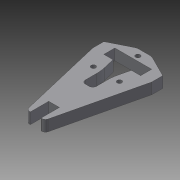
# Autodesk Inventor part: Vert Moto Mount skinny
Saved by Autodesk Inventor 2015 (Build 190159000, 159)
## iProperties
Created: 2012-05-11
Part Number: Vert Moto Mount skinny
Material: Generic
Document SubType Name: Modeling
Designer: user
Density: 1 g/cm^3
Appearance: Default
Author: user
Autodesk Inventor part; units mm, degrees
ref_plane "YZ Plane" through (0, 0, 0) normal (1, 0, 0) x (0, 1, 0)
ref_plane "XZ Plane" through (0, 0, 0) normal (0, 1, 0) x (-1, 0, 0)
ref_plane "XY Plane" through (0, 0, 0) normal (0, 0, 1) x (1, 0, 0)
sketch "Sketch1" plane through (0, 0, 0) normal (0, 0, 1) x (1, 0, 0)
  circle A0 centre (0, 35.5) radius 10 construction
  line L0 (-2.9, -10) -> (-2.9, 0)
  line L1 (-2.9, 0) -> (2.9, 0)
  line L2 (2.9, 0) -> (2.9, -10)
  line L3 (-3.3173, -10) -> (-2.9, -10)
  line L4 (2.9, -10) -> (3.3173, -10)
  circle A1 centre (-7.0711, 28.4289) radius 1.25
  circle A2 centre (7.0711, 28.4289) radius 1.25
  circle A3 centre (0, 45.5) radius 1.25
  line L5 (-16, 37) -> (-16, 43)
  line L6 (16, 37) -> (16, 43)
  line L7 (-5.2638, -8.4597) -> (-16, 37)
  line L8 (5.2638, -8.4597) -> (16, 37)
  line L9 (-16, 43) -> (-4.8446, 48.5777)
  line L10 (-3.0557, 49) -> (3.0557, 49)
  line L11 (4.8446, 48.5777) -> (16, 43)
  arc A4 (-3.0557, 49) -> (-4.8446, 48.5777) centre (-3.0557, 45) ccw
  arc A5 (4.8446, 48.5777) -> (3.0557, 49) centre (3.0557, 45) ccw
  line L12 (0, 49) -> (0, 0) construction
  line L13 (-7.0711, 28.4289) -> (0, 35.5) construction
  line L14 (0, 35.5) -> (7.0711, 28.4289) construction
  arc A6 (-5.2638, -8.4597) -> (-3.3173, -10) centre (-3.3173, -8) ccw
  arc A7 (3.3173, -10) -> (5.2638, -8.4597) centre (3.3173, -8) ccw
  circle A8 centre (0, 35.5) radius 15.25 construction
  point P0 (0, 43)
  point P1 (4.9, -10)
  point P2 (-4.9, -10)
  point P3 (0, 43)
  point P4 (-4, 49)
  point P5 (4, 49)
  dimension "d69" = 20
  dimension "d88" = 5.8
  dimension "d95" = 2
  dimension "d96" = 2
  dimension "d97" = 10
  dimension "d98" = 10
  dimension "d109" = 43
  dimension "d112" = 2.5
  dimension "d113" = 2.5
  dimension "d114" = 2.5
  dimension "d123" = 32
  dimension "d126" = 8
  dimension "d127" = 4
  dimension "d144" = 16
  dimension "d145" = 35.5
  dimension "d153" = 6
  dimension "d155" = 6
  dimension "d156" = 135
  dimension "d163" = 2
  dimension "d169" = 30.5
  constraints: 30 end point, 12 point on circle, 9 centre point, 8 point on line, 8 tangent, 5 coincident, 5 perpendicular, 4 horizontal alignment, 4 vertical alignment, 2 equal length, 2 equal radius, 2 midpoint, 1 horizontal, 1 vertical
  measures "d69" diameter of A0
  measures "d88" distance of L0.end L1.end
  measures "d95" distance of point (-4.9, -10) L0.start
  measures "d96" distance of L2.end point (4.9, -10)
  measures "d97" distance between parallel lines of L3 L1
  measures "d98" distance between parallel lines of L1 L4
  measures "d109" distance from line of L1 point (0, 43)
  measures "d112" diameter of A2
  measures "d113" diameter of A1
  measures "d114" diameter of A3
  measures "d123" distance between parallel lines of L6 L5
  measures "d126" distance of point (-4, 49) point (4, 49)
  measures "d127" radius of A4
  measures "d144" distance from line of L13.end L6
  measures "d145" distance from line of L1 L13.end
  measures "d153" distance of L5.start L5.end
  measures "d155" distance from line of L5.end L10
  measures "d156" angle of L12 L13
  measures "d163" radius of A6
  measures "d169" diameter of A8
extrude "Extrusion7" add sketch "Sketch1" along normal blind 6
sketch "Sketch3" plane through (0, 0, 6) normal (0, 0, 1) x (1, 0, 0)
  line L0 (16, 37) -> (16, 43) projected
  line L1 (-16, 43) -> (-16, 37) projected
  line L2 (-10, 43) -> (10, 43)
  line L3 (10, 43) -> (10, 37)
  line L4 (-10, 37) -> (-10, 43)
  line L5 (10, 37) -> (5, 37)
  line L6 (-5, 37) -> (-10, 37)
  line L7 (5.2638, -8.4597) -> (16, 37) projected
  line L8 (-16, 37) -> (-5.2638, -8.4597) projected
  circle A0 centre (0, 45.5) radius 1.25 projected
  circle A1 centre (7.0711, 28.4289) radius 1.25 projected
  circle A2 centre (-7.0711, 28.4289) radius 1.25 projected
  line L9 (3.0557, 49) -> (-3.0557, 49) projected
  line L10 (0, 45.5) -> (0, 35.4997) construction
  line L11 (-7.0711, 28.4289) -> (0, 35.5003) construction
  line L12 (7.0711, 28.4289) -> (0, 35.4997) construction
  line L13 (-5, 37) -> (-3.5355, 30.7988)
  line L14 (-3, 26.2019) -> (-3, 20)
  line L15 (-1, 18) -> (1, 18)
  line L16 (3, 20) -> (3, 26.2019)
  line L17 (3.5355, 30.7988) -> (5, 37)
  arc A3 (-3, 26.2019) -> (-3.5355, 30.7988) centre (-23, 26.2019) ccw
  arc A4 (3.5355, 30.7988) -> (3, 26.2019) centre (23, 26.2019) ccw
  arc A5 (-3, 20) -> (-1, 18) centre (-1, 20) ccw
  arc A6 (1, 18) -> (3, 20) centre (1, 20) ccw
  point P0 (0, 0)
  point P1 (4.9, -10)
  point P2 (-4.9, -10)
  point P3 (0, 18)
  dimension "d132" = 6
  dimension "d134" = 6
  dimension "d135" = 6
  dimension "d148" = 5
  dimension "d149" = 5
  dimension "d157" = 25
  dimension "d160" = 6
  dimension "d161" = 20
  dimension "d162" = 2
  constraints: 26 end point, 8 point on circle, 8 tangent, 5 parallel, 5 perpendicular, 4 centre point, 2 equal radius, 2 horizontal alignment, 1 horizontal, 1 midpoint, 1 point on line, 1 vertical, 1 vertical alignment
  measures "d132" distance of L2.end L3.end
  measures "d134" distance between parallel lines of L1 L4
  measures "d135" distance between parallel lines of L0 L3
  measures "d148" distance of L6.start L4.start
  measures "d149" distance of L3.end L5.end
  measures "d157" distance between parallel lines of L2 L15
  measures "d160" distance between parallel lines of L16 L14
  measures "d161" radius of A3
  measures "d162" radius of A5
extrude "Extrusion8" cut sketch "Sketch3" against normal through all contours L2 L3 L5 L17 A4 L16 A6 L15 A5 L14 A3 L13 L6 L4
body "Solid7"
